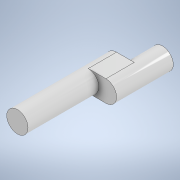
# Autodesk Inventor part: 偏心支轴
Saved by Autodesk Inventor 2022 (Build 260153000, 153)
## iProperties
Created: 2022-05-22
Part Number: 偏心支轴
Material: 常规
Document SubType Name: Modeling
Designer: zhcne
Density: 1 g/cm^3
Appearance: 默认
Author: zhcne
Autodesk Inventor part; units mm, degrees
ref_plane "YZ Plane" through (0, 0, 0) normal (1, 0, 0) x (0, 1, 0)
ref_plane "XZ Plane" through (0, 0, 0) normal (0, 1, 0) x (-1, 0, 0)
ref_plane "XY Plane" through (0, 0, 0) normal (0, 0, 1) x (1, 0, 0)
sketch "草图1" plane through (0, 0, 0) normal (0, 0, 1) x (1, 0, 0)
  circle A0 centre (0, 0) radius 1.5
  dimension "d0" = 3
  constraints: 1 centre point, 1 coincident
  measures "d0" diameter of A0
extrude "拉伸1" add sketch "草图1" along normal blind 4
sketch "草图2" plane through (0, 0, 4) normal (0, 0, 1) x (1, 0, 0)
  arc A0 (0, -1.5) -> (0, 1.5) centre (0, 0) ccw
  circle A1 centre (0, 0) radius 1.5 projected
  line L0 (0, -1.5) -> (-2.5, -1.5)
  line L1 (0, 1.5) -> (-2.5, 1.5)
  line L2 (-2.5, 1.5) -> (-2.5, -1.5)
  arc A2 (-2.5, 1.5) -> (-2.5, -1.5) centre (-2.5, 0) ccw
  dimension "d3" = 2.5
  constraints: 6 end point, 6 point on circle, 5 tangent, 2 centre point, 2 horizontal, 1 coincident, 1 midpoint, 1 perpendicular
  measures "d3" distance of L0.start L0.end
extrude "拉伸2" add sketch "草图2" along normal blind 4
sketch "草图3" plane through (0, 0, 8) normal (0, 0, 1) x (1, 0, 0)
  arc A0 (-2.5, 1.5) -> (-2.5, -1.5) centre (-2.5, 0) ccw projected
  circle A1 centre (-2.5, 0) radius 1.5
  point P0 (0, 0)
  constraints: 1 centre point, 1 coincident
extrude "拉伸3" add sketch "草图3" along normal blind 10
